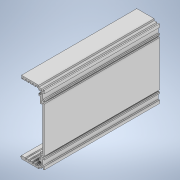
# Autodesk Inventor part: Fischer HB
Saved by Autodesk Inventor 2021.4 (Build 254397000, 397)
## iProperties
Created: 2019-10-29
Part Number: Fischer HB
Material: Generic
Document SubType Name: Modeling
Designer: test
Density: 1 g/cm^3
Appearance: Default
Author: test
Autodesk Inventor part; units mm, degrees
ref_plane "YZ Plane" through (0, 0, 0) normal (1, 0, 0) x (0, 1, 0)
ref_plane "XZ Plane" through (0, 0, 0) normal (0, 1, 0) x (-1, 0, 0)
ref_plane "XY Plane" through (0, 0, 0) normal (0, 0, 1) x (1, 0, 0)
sketch "Sketch1" plane through (0, 0, 0) normal (0, 0, 1) x (1, 0, 0)
  line L0 (0, 52.5) -> (25.1, 52.5)
  line L1 (33.1, 32.75) -> (33.1, -32.75)
  line L2 (0, -48.25) -> (5.56, -48.25)
  line L3 (27, -30.7) -> (30.6, -30.7)
  line L4 (30.6, -30.7) -> (30.6, 30.7)
  line L5 (30.6, 30.7) -> (27, 30.7)
  line L6 (25.1, 48.35) -> (22.6, 48.35)
  arc A0 (-0.95, -49.45) -> (-0.95, -50.75) centre (-0.95, -50.1) ccw
  line L7 (-0.95, -49.45) -> (0, -49.45)
  line L8 (0, -49.45) -> (0, -48.25)
  line L9 (-0.95, -50.75) -> (0, -50.75)
  line L10 (0, -50.75) -> (0, -52.5)
  line L11 (0, -52.5) -> (25.1, -52.5)
  line L12 (25.1, -52.5) -> (25.1, -50)
  line L13 (25.1, -50) -> (29, -50)
  line L14 (29, -50) -> (29, -47.55)
  line L15 (29, -47.55) -> (31.5, -47.55)
  line L16 (31.5, -47.55) -> (31.5, -50)
  line L17 (31.5, -50) -> (33.1, -50)
  line L18 (25.1, 52.5) -> (25.1, 50)
  line L19 (25.1, 50) -> (29, 50)
  line L20 (29, 50) -> (29, 47.55)
  line L21 (29, 47.55) -> (31.5, 47.55)
  line L22 (31.5, 47.55) -> (31.5, 50)
  line L23 (31.5, 50) -> (33.1, 50)
  arc A1 (1.85, 49.45) -> (1.85, 50.95) centre (1.85, 50.2) ccw
  line L24 (0, 49.45) -> (0, 48.35)
  line L25 (0, 50.95) -> (0, 52.5)
  line L26 (1.85, 50.95) -> (0, 50.95)
  line L27 (1.85, 49.45) -> (0, 49.45)
  line L28 (27, 30.7) -> (27, 39.7)
  line L29 (27, 39.7) -> (25.1, 39.7)
  line L30 (25.1, 46.25) -> (25.1, 48.35)
  line L31 (27, -30.7) -> (27, -39.7)
  line L32 (27, -39.7) -> (25.1, -39.7)
  line L33 (25.1, -46.25) -> (25.1, -48.25)
  line L34 (-8.54, 0) -> (40.04, 0) projected
  line L35 (33.1, 50) -> (33.1, 45.6)
  line L36 (33.1, 45.6) -> (31.1, 45.6)
  line L37 (31.1, 45.6) -> (31.1, 37.6)
  line L38 (31.1, 37.6) -> (33.1, 37.6)
  line L39 (33.1, -37.6) -> (31.1, -37.6)
  line L40 (31.1, -37.6) -> (31.1, -45.6)
  line L41 (31.1, -45.6) -> (33.1, -45.6)
  line L42 (33.1, -45.6) -> (33.1, -50)
  line L43 (33.1, 37.6) -> (33.1, 35.75)
  line L44 (33.1, 35.75) -> (30.55, 34.25)
  line L45 (30.55, 34.25) -> (33.1, 32.75)
  line L46 (33.1, -32.75) -> (30.55, -34.25)
  line L47 (30.55, -34.25) -> (33.1, -35.75)
  line L48 (33.1, -35.75) -> (33.1, -37.6)
  line L49 (22.6, 48.35) -> (22.6, 50.2)
  line L50 (22.6, 50.2) -> (20.8, 50.2)
  line L51 (20.8, 50.2) -> (20.8, 48.35)
  line L52 (20.8, 48.35) -> (17.52, 48.35)
  line L53 (17.52, 48.35) -> (17.52, 50.2)
  line L54 (17.52, 50.2) -> (15.72, 50.2)
  line L55 (15.72, 50.2) -> (15.72, 48.35)
  line L56 (15.72, 48.35) -> (12.44, 48.35)
  line L57 (12.44, 48.35) -> (12.44, 50.2)
  line L58 (12.44, 50.2) -> (10.64, 50.2)
  line L59 (10.64, 50.2) -> (10.64, 48.35)
  line L60 (10.64, 48.35) -> (7.36, 48.35)
  line L61 (7.36, 48.35) -> (7.36, 50.2)
  line L62 (7.36, 50.2) -> (5.56, 50.2)
  line L63 (5.56, 50.2) -> (5.56, 48.35)
  line L64 (5.56, 48.35) -> (0, 48.35)
  line L65 (5.56, -48.25) -> (5.56, -50.2)
  line L66 (5.56, -50.2) -> (7.36, -50.2)
  line L67 (7.36, -50.2) -> (7.36, -48.25)
  line L68 (7.36, -48.25) -> (10.64, -48.25)
  line L69 (10.64, -48.25) -> (10.64, -50.2)
  line L70 (10.64, -50.2) -> (12.44, -50.2)
  line L71 (12.44, -50.2) -> (12.44, -48.25)
  line L72 (12.44, -48.25) -> (15.72, -48.25)
  line L73 (15.72, -48.25) -> (15.72, -50.2)
  line L74 (15.72, -50.2) -> (17.52, -50.2)
  line L75 (17.52, -50.2) -> (17.52, -48.25)
  line L76 (17.52, -48.25) -> (20.8, -48.25)
  line L77 (20.8, -48.25) -> (20.8, -50.2)
  line L78 (20.8, -50.2) -> (22.6, -50.2)
  line L79 (22.6, -50.2) -> (22.6, -48.25)
  line L80 (22.6, -48.25) -> (25.1, -48.25)
  line L81 (25.1, 42.65) -> (25.1, 39.7)
  line L82 (25.1, 42.65) -> (25.85, 42.65)
  line L83 (25.85, 42.65) -> (25.85, 41.8)
  line L84 (25.85, 41.8) -> (27.55, 41.8)
  line L85 (27.55, 41.8) -> (27.55, 42.65)
  line L86 (27.55, 42.65) -> (28.6, 42.65)
  line L87 (28.6, 42.65) -> (28.6, 46.25)
  line L88 (28.6, 46.25) -> (27.55, 46.25)
  line L89 (27.55, 46.25) -> (27.55, 47.1)
  line L90 (27.55, 47.1) -> (25.85, 47.1)
  line L91 (25.85, 47.1) -> (25.85, 46.25)
  line L92 (25.85, 46.25) -> (25.1, 46.25)
  line L93 (25.1, -46.25) -> (25.85, -46.25)
  line L94 (25.85, -46.25) -> (25.85, -47.1)
  line L95 (25.85, -47.1) -> (27.55, -47.1)
  line L96 (27.55, -47.1) -> (27.55, -46.25)
  line L97 (27.55, -46.25) -> (28.6, -46.25)
  line L98 (28.6, -46.25) -> (28.6, -42.65)
  line L99 (28.6, -42.65) -> (27.55, -42.65)
  line L100 (27.55, -42.65) -> (27.55, -41.8)
  line L101 (27.55, -41.8) -> (25.85, -41.8)
  line L102 (25.85, -41.8) -> (25.85, -42.65)
  line L103 (25.85, -42.65) -> (25.1, -42.65)
  line L104 (25.1, -42.65) -> (25.1, -39.7)
  point P0 (0, 0)
  dimension "d7" = 21.8
  dimension "d10" = 0.65
  dimension "d11" = 34.7
  dimension "d14" = 105
  dimension "d16" = 100
  dimension "d17" = 95.1
  dimension "d18" = 2.5
  dimension "d20" = 1.6
  dimension "d24" = 2.5
  dimension "d29" = 96.6
  dimension "d30" = 1.85
  dimension "d31" = 1.5
  dimension "d32" = 100.3
  dimension "d33" = 8
  dimension "d34" = 33.1
  dimension "d35" = 2.6
  dimension "d36" = 12.8
  dimension "d37" = 6.1
  dimension "d49" = 8
  dimension "d50" = 4.4
  dimension "d51" = 4.1
  dimension "d52" = 3
  dimension "d53" = 2.55
  dimension "d55" = 68.5
  dimension "d56" = 1.8
  dimension "d57" = 5.08
  dimension "d58" = 10.5
  dimension "d59" = 4.15
  dimension "d60" = 3.6
  dimension "d61" = 0.75
  dimension "d62" = 1.7
  dimension "d63" = 3.5
  dimension "d64" = 5.3
  dimension "d65" = 94.2
  constraints: 210 end point, 59 perpendicular, 37 point on line, 24 collinear, 15 equal length, 10 vertical, 10 vertical alignment, 9 horizontal, 4 point on circle, 2 centre point, 2 parallel, 1 horizontal alignment, 10 other
  measures "d7" distance between parallel lines of L0 L5
  measures "d10" radius of A0
  measures "d14" distance between parallel lines of L11 L0
  measures "d16" distance between parallel lines of L13 L19
  measures "d17" distance between parallel lines of L21 L15
  measures "d18" distance of L20.end L21.end
  measures "d20" distance of L16.end L17.end
  measures "d24" distance between parallel lines of L1 L4
  measures "d29" distance between parallel lines of L2 L6
  measures "d30" distance from line of L2 A0.centre
  measures "d31" distance of L26.start L27.start
  measures "d32" vertical distance of A0.centre A1.centre
  measures "d33" distance between parallel lines of L1 L18
  measures "d34" distance between parallel lines of L25 L1
  measures "d36" distance between parallel lines of L0 L29
  measures "d37" distance between parallel lines of L1 L28
  measures "d49" distance of L36.end L37.end
  measures "d50" distance of L23.end L35.end
  measures "d51" distance between parallel lines of L37 L28
  measures "d52" distance of L1.start L43.end
  measures "d53" distance from line of L1 L44.end
  measures "d55" distance of L44.end L46.end
  measures "d56" distance of L49.end L50.end
  measures "d57" distance between parallel lines of L59 L63
  measures "d58" distance between parallel lines of L35 L49
  measures "d59" distance between parallel lines of L64 L0
  measures "d60" distance of L30.start L81.start
  measures "d61" distance of L81.start L82.end
  measures "d62" distance of L83.end L84.end
  measures "d63" distance between parallel lines of L30 L87
  measures "d64" distance between parallel lines of L84 L90
  measures "d65" distance between parallel lines of L90 L95
extrude "Extrusion1" add sketch "Sketch1" along normal blind 167.2
sketch "Sketch2" plane through (0, 0, 167.2) normal (0, 0, 1) x (1, 0, 0)
  line L0 (33.1, -50) -> (33.1, 50) projected
  line L1 (-8.54, 0) -> (40.04, 0) projected
  point P0 (0, 0)
  point P1 (30.55, 34.25)
  point P2 (30.55, -34.25)
  dimension "d40" = 2.55
  dimension "d41" = 68.5
  constraints: 1 symmetric about line, 1 vertical alignment
  measures "d40" distance from line of L0 point (30.55, 34.25)
  measures "d41" distance of point (30.55, -34.25) point (30.55, 34.25)
hole "Hole1" at (30.55, -34.25, 167.2) at (30.55, 34.25, 167.2) direction (0, 0, -1) diameter 3 end through all
body "Solid1"
